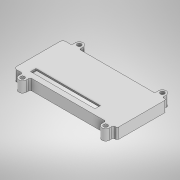
# Autodesk Inventor part: frontpackCOVER2
Saved by Autodesk Inventor 2021 (Build 250183000, 183)
## iProperties
Created: 2021-09-03
Part Number: frontpackCOVER2
Material: Generic
Document SubType Name: Modeling
Designer: perez
Density: 1 g/cm^3
Appearance: Default
Author: perez
Autodesk Inventor part; units mm, degrees
ref_plane "YZ Plane" through (0, 0, 0) normal (1, 0, 0) x (0, 1, 0)
ref_plane "XZ Plane" through (0, 0, 0) normal (0, 1, 0) x (-1, 0, 0)
ref_plane "XY Plane" through (0, 0, 0) normal (0, 0, 1) x (1, 0, 0)
sketch "Sketch1" plane through (0, 0, 0) normal (0, 1, 0) x (-1, 0, 0)
  line L0 (0, 0) -> (37, 0) construction
  line L1 (37, 0) -> (37, -30) construction
  line L2 (37, -30) -> (0, -30) construction
  line L3 (0, -30) -> (0, 0) construction
  line L4 (75.5, -6) -> (38, -6) construction
  line L5 (38, -6) -> (38, -24) construction
  line L6 (38, -24) -> (75.5, -24) construction
  line L7 (75.5, -24) -> (75.5, -6) construction
  line L8 (94, 0) -> (76.5, 0) construction
  line L9 (76.5, 0) -> (76.5, -28) construction
  line L10 (76.5, -28) -> (94, -28) construction
  line L11 (94, -28) -> (94, 0) construction
  line L12 (-1, 1) -> (117.5, 1)
  line L13 (117.5, 1) -> (117.5, -31)
  line L14 (117.5, -31) -> (-1, -31)
  line L15 (-1, -31) -> (-1, 1)
  line L16 (0, 0) -> (94, 0)
  line L17 (94, 0) -> (94, -30)
  line L18 (94, -30) -> (0, -30)
  line L19 (0, -30) -> (0, 0)
  line L20 (38, -8) -> (37, -8)
  line L21 (37, -8) -> (37, -22)
  line L22 (37, -22) -> (38, -22)
  line L23 (38, -22) -> (38, -8)
  line L24 (73.5, -6) -> (40, -6)
  line L25 (40, -6) -> (40, -5)
  line L26 (40, -5) -> (73.5, -5)
  line L27 (73.5, -5) -> (73.5, -6)
  line L28 (73.5, -24) -> (40, -24)
  line L29 (40, -24) -> (40, -25)
  line L30 (40, -25) -> (73.5, -25)
  line L31 (73.5, -25) -> (73.5, -24)
  line L32 (76.5, -8) -> (75.5, -8)
  line L33 (75.5, -8) -> (75.5, -22)
  line L34 (75.5, -22) -> (76.5, -22)
  line L35 (76.5, -22) -> (76.5, -8)
  line L36 (115, -31) -> (115, -33.5) construction
  line L37 (58.25, -31) -> (58.25, -33.5) construction
  line L38 (4, -31) -> (4, -33.5) construction
  line L39 (115, 1) -> (115, 3.5) construction
  line L40 (58.25, 1) -> (58.25, 3.5) construction
  line L41 (4, 1) -> (4, 3.5) construction
  circle A0 centre (115, -33.5) radius 2.5
  circle A1 centre (58.25, -33.5) radius 2.5
  circle A2 centre (4, -33.5) radius 2.5
  circle A3 centre (4, 3.5) radius 2.5
  circle A4 centre (58.25, 3.5) radius 2.5
  circle A5 centre (115, 3.5) radius 2.5
  line L42 (117.5, 1) -> (117.5, 3.5)
  line L43 (112.5, 3.5) -> (112.5, 1)
  line L44 (60.75, 3.5) -> (60.75, 1)
  line L45 (55.75, 3.5) -> (55.75, 1)
  line L46 (6.5, 3.5) -> (6.5, 1)
  line L47 (1.5, 3.5) -> (1.5, 1)
  line L48 (1.5, -33.5) -> (1.5, -31)
  line L49 (6.5, -33.5) -> (6.5, -31)
  line L50 (55.75, -33.5) -> (55.75, -31)
  line L51 (60.75, -33.5) -> (60.75, -31)
  line L52 (117.5, -33.5) -> (117.5, -31)
  line L53 (112.5, -33.5) -> (112.5, -31)
  circle A6 centre (115, -33.5) radius 1.55
  circle A7 centre (58.25, -33.5) radius 1.55
  circle A8 centre (4, -33.5) radius 1.55
  circle A9 centre (4, 3.5) radius 1.55
  circle A10 centre (58.25, 3.5) radius 1.55
  circle A11 centre (115, 3.5) radius 1.55
  line L54 (57.75, -30) -> (58.75, -30)
  line L55 (58.75, -30) -> (58.75, -25)
  line L56 (58.75, -25) -> (57.75, -25)
  line L57 (57.75, -25) -> (57.75, -30)
  line L58 (57.75, -5) -> (58.75, -5)
  line L59 (58.75, -5) -> (58.75, 0)
  line L60 (58.75, 0) -> (57.75, 0)
  line L61 (57.75, 0) -> (57.75, -5)
  line L62 (40, -25) -> (41, -25)
  line L63 (41, -25) -> (41, -30)
  line L64 (41, -30) -> (40, -30)
  line L65 (40, -30) -> (40, -25)
  line L66 (40, -5) -> (41, -5)
  line L67 (41, -5) -> (41, 0)
  line L68 (41, 0) -> (40, 0)
  line L69 (40, 0) -> (40, -5)
  line L70 (73.5, -5) -> (72.5, -5)
  line L71 (72.5, -5) -> (72.5, 0)
  line L72 (72.5, 0) -> (73.5, 0)
  line L73 (73.5, 0) -> (73.5, -5)
  line L74 (73.5, -25) -> (72.5, -25)
  line L75 (72.5, -25) -> (72.5, -30)
  line L76 (72.5, -30) -> (73.5, -30)
  line L77 (73.5, -30) -> (73.5, -25)
  dimension "d0" = 37
  dimension "d1" = 30
  dimension "d2" = 18
  dimension "d3" = 37.5
  dimension "d4" = 1
  dimension "d5" = 6
  dimension "d6" = 17.5
  dimension "d7" = 28
  dimension "d8" = 1
  dimension "d9" = 1
  dimension "d10" = 1
  dimension "d11" = 1
  dimension "d12" = 117.5
  dimension "d13" = 2
  dimension "d14" = 2
  dimension "d15" = 1
  dimension "d16" = 1
  dimension "d17" = 2
  dimension "d18" = 2
  dimension "d19" = 2
  dimension "d20" = 2
  dimension "d21" = 2.5
  dimension "d22" = 2.5
  dimension "d23" = 5
  dimension "d24" = 2.5
  dimension "d25" = 2.5
  dimension "d26" = 2.5
  dimension "d27" = 2.5
  dimension "d28" = 5
  dimension "d29" = 5
  dimension "d30" = 2.5
  dimension "d31" = 3.1
  dimension "d32" = 3.1
  dimension "d33" = 3.1
  dimension "d34" = 3.1
  dimension "d35" = 3.1
  dimension "d36" = 3.1
  dimension "d44" = 1
  dimension "d45" = 1
  dimension "d46" = 0.5
  dimension "d47" = 0
  dimension "d48" = 1
  dimension "d49" = 1
  dimension "d50" = 1
  dimension "d51" = 1
  constraints: 152 end point, 30 parallel, 24 point on line, 16 point on circle, 15 perpendicular, 14 horizontal, 12 centre point, 12 coincident, 12 vertical, 8 tangent, 22 other
  measures "d0" distance of L1.end L2.end
  measures "d1" distance of L0.end L1.end
  measures "d2" distance of L4.end L5.end
  measures "d3" distance of L5.end L6.end
  measures "d4" distance between parallel lines of L1 L5
  measures "d5" distance between parallel lines of L2 L6
  measures "d6" distance of L10.end L9.end
  measures "d7" distance of L9.end L8.end
  measures "d8" distance between parallel lines of L7 L9
  measures "d9" distance between parallel lines of L15 L3
  measures "d12" distance between parallel lines of L13 L3
  measures "d13" distance between parallel lines of L20 L4
  measures "d14" distance between parallel lines of L22 L6
  measures "d15" distance of L30.end L28.start
  measures "d16" distance of L26.end L24.start
  measures "d17" distance between parallel lines of L5 L25
  measures "d18" distance between parallel lines of L7 L27
  measures "d19" distance between parallel lines of L6 L34
  measures "d20" distance between parallel lines of L4 L32
  measures "d21" distance of L36.start L36.end
  measures "d22" distance between parallel lines of L13 L36
  measures "d23" distance between parallel lines of L15 L38
  measures "d24" distance of L37.start L37.end
  measures "d25" distance of L39.start L39.end
  measures "d26" distance of L40.start L40.end
  measures "d27" distance of L41.start L41.end
  measures "d28" diameter of A0
  measures "d29" diameter of A1
  measures "d30" distance of L38.start L38.end
  measures "d31" diameter of A6
  measures "d32" diameter of A7
  measures "d33" diameter of A8
  measures "d34" diameter of A9
  measures "d35" diameter of A10
  measures "d36" diameter of A11
  measures "d44" distance between parallel lines of L55 L57
  measures "d45" distance between parallel lines of L59 L61
  measures "d46" distance between parallel lines of L37 L57
  measures "d47" distance between parallel lines of L40 L37
  measures "d48" distance of L63.end L64.end
  measures "d49" distance of L68.end L67.end
  measures "d50" distance of L71.end L72.end
  measures "d51" distance of L76.end L75.end
extrude "Extrusion1" add sketch "Sketch1" along normal blind 7 contours L12 L13 L14 L15 | L47 A3 L12 | A3 L46 L12 | A3 | L14 A2 L48 | L14 L49 A2 | A2 | L45 A4 L12 | A4 L44 L12 | A4 | L14 A1 L50 | L14 L51 A1 | A1 | L43 A5 L12 | A5 L42 L12 | A5 | L14 A0 L53 | L14 L52 A0 | A0 | L16 L67 L26 L69 | L26 L27 L24 L25 | L65 L30 L63 L18 | L16 L59 L26 L61 | L29 L28 L31 L30 | L57 L30 L55 L18 | L16 L73 L26 L71 | L75 L30 L77 L18 | L23 L22 L21 L20 | L35 L34 L33 L32
sketch "Sketch2" plane through (0, 0, 0) normal (0, -1, 0) x (1, 0, 0)
  line L0 (-117.5, -33.5) -> (-117.5, 3.5) projected
  arc A0 (-117.5, -33.5) -> (-112.5, -33.5) centre (-115, -33.5) ccw projected
  line L1 (-112.5, -31) -> (-112.5, -33.5) projected
  line L2 (-60.75, -31) -> (-112.5, -31) projected
  line L3 (-60.75, -33.5) -> (-60.75, -31) projected
  arc A1 (-60.75, -33.5) -> (-55.75, -33.5) centre (-58.25, -33.5) ccw projected
  line L4 (-55.75, -31) -> (-55.75, -33.5) projected
  line L5 (-6.5, -31) -> (-55.75, -31) projected
  line L6 (-6.5, -33.5) -> (-6.5, -31) projected
  arc A2 (-6.5, -33.5) -> (-1.5, -33.5) centre (-4, -33.5) ccw projected
  line L7 (-1.5, -31) -> (-1.5, -33.5) projected
  line L8 (1, -31) -> (-1.5, -31) projected
  line L9 (1, 1) -> (1, -31) projected
  line L10 (-1.5, 1) -> (1, 1) projected
  line L11 (-1.5, 3.5) -> (-1.5, 1) projected
  arc A3 (-1.5, 3.5) -> (-6.5, 3.5) centre (-4, 3.5) ccw projected
  line L12 (-6.5, 1) -> (-6.5, 3.5) projected
  line L13 (-55.75, 1) -> (-6.5, 1) projected
  line L14 (-55.75, 3.5) -> (-55.75, 1) projected
  arc A4 (-55.75, 3.5) -> (-60.75, 3.5) centre (-58.25, 3.5) ccw projected
  line L15 (-60.75, 1) -> (-60.75, 3.5) projected
  line L16 (-112.5, 1) -> (-60.75, 1) projected
  line L17 (-112.5, 3.5) -> (-112.5, 1) projected
  arc A5 (-112.5, 3.5) -> (-117.5, 3.5) centre (-115, 3.5) ccw projected
  circle A6 centre (-58.25, 3.5) radius 1.55 projected
  circle A7 centre (-4, 3.5) radius 1.55 projected
  circle A8 centre (-4, -33.5) radius 1.55 projected
  circle A9 centre (-58.25, -33.5) radius 1.55 projected
  circle A10 centre (-115, 3.5) radius 1.55 projected
  circle A11 centre (-115, -33.5) radius 1.55 projected
  line L18 (-41, 0) -> (-57.75, 0) projected
  line L19 (0, -30) -> (0, 0) projected
  line L20 (-57.75, -30) -> (-41, -30) projected
  line L21 (-94, 0) -> (-94, -30) projected
  line L22 (-41, -5) -> (-41, 0) projected
  line L23 (-57.75, -5) -> (-41, -5) projected
  line L24 (-57.75, 0) -> (-57.75, -5) projected
  line L25 (-41, -30) -> (-41, -25) projected
  line L26 (-57.75, -25) -> (-57.75, -30) projected
  line L27 (-41, -25) -> (-57.75, -25) projected
  line L28 (-72.5, -25) -> (-72.5, -30) projected
  line L29 (-58.75, -25) -> (-72.5, -25) projected
  line L30 (-58.75, -30) -> (-58.75, -25) projected
  line L31 (-72.5, -30) -> (-58.75, -30) projected
  line L32 (-72.5, 0) -> (-72.5, -5) projected
  line L33 (-58.75, 0) -> (-72.5, 0) projected
  line L34 (-58.75, -5) -> (-58.75, 0) projected
  line L35 (-72.5, -5) -> (-58.75, -5) projected
  line L36 (-73.5, 0) -> (-94, 0) projected
  line L37 (-73.5, -6) -> (-73.5, 0) projected
  line L38 (-40, -6) -> (-73.5, -6) projected
  line L39 (-40, 0) -> (-40, -6) projected
  line L40 (0, 0) -> (-40, 0) projected
  line L41 (-40, -30) -> (0, -30) projected
  line L42 (-40, -24) -> (-40, -30) projected
  line L43 (-73.5, -24) -> (-40, -24) projected
  line L44 (-73.5, -30) -> (-73.5, -24) projected
  line L45 (-94, -30) -> (-73.5, -30) projected
extrude "Extrusion2" add sketch "Sketch2" along normal blind 1 contours L0 A5 L17 L16 L15 A4 L14 L13 L12 A3 L11 L10 L9 L8 L7 A2 L6 L5 L4 A1 L3 L2 L1 A0 | L22 L23 L24 L18 | L41 L42 L43 L44 L45 L21 L36 L37 L38 L39 L40 L19 | L26 L27 L25 L20 | L29 L30 L31 L28 | L33 L34 L35 L32
fillet "Fillet2" radius 1 32 edges at (-73.5, 3.5, -6) (-73.5, 3.5, -24) (-40, 3.5, -24) (1, 3, -31) (-1.5, 3, -31) (1, 3, 1) (-55.75, 3, -31) (-1.5, 3, 1) (-55.75, 3, 1) (-112.5, 3, 1) (-112.5, 3, -31) (-60.75, 3, -31) (-6.5, 3, -31) (-60.75, 3, 1) (-6.5, 3, 1) (-40, 3.5, -6) (-72.5, 3.5, 0) (-57.75, 3.5, 0) (-72.5, 3.5, -25) (-57.75, 3.5, -25) (-41, 3.5, -25) (-58.75, 3.5, -25) (-41, 3.5, 0) (-58.75, 3.5, 0) (-72.5, 3.5, -30) (-57.75, 3.5, -30) (-57.75, 3.5, -5) (-72.5, 3.5, -5) (-41, 3.5, -5) (-58.75, 3.5, -5) (-58.75, 3.5, -30) (-41, 3.5, -30)
sketch "Sketch5" plane through (0, 7, 0) normal (0, 1, 0) x (1, 0, 0)
  line L0 (-120.447, 38.9055) -> (3.6698, 38.9055)
  line L1 (3.6698, 38.9055) -> (3.6698, -10.7705)
  line L2 (3.6698, -10.7705) -> (-120.447, -10.7705)
  line L3 (-120.447, -10.7705) -> (-120.447, 38.9055)
  point P0 (0, 0)
  constraints: 8 end point, 2 parallel, 1 horizontal, 1 perpendicular
extrude "Extrusion5" cut sketch "Sketch5" against normal blind 7
sketch "Sketch13" plane through (0, 0, 0) normal (0, 1, 0) x (1, 0, 0)
  line L0 (-64.5, 29) -> (-1, 29)
  line L1 (-1, 29) -> (-1, 1)
  line L2 (-1, 1) -> (-64.5, 1)
  line L3 (-64.5, 1) -> (-64.5, 29)
  line L4 (1, 30) -> (1, 0) projected
  line L5 (-54.75, 31) -> (-7.5, 31) projected
  line L6 (-7.5, -1) -> (-54.75, -1) projected
  line L7 (-117.5, -3.5) -> (-117.5, 33.5) projected
  line L8 (-77.5, 28.5) -> (-67.5, 28.5)
  line L9 (-67.5, 28.5) -> (-67.5, 21.5)
  line L10 (-67.5, 21.5) -> (-77.5, 21.5)
  line L11 (-77.5, 21.5) -> (-77.5, 28.5)
  line L12 (-77.5, 11) -> (-67.5, 11)
  line L13 (-67.5, 11) -> (-67.5, 4)
  line L14 (-67.5, 4) -> (-77.5, 4)
  line L15 (-77.5, 4) -> (-77.5, 11)
  line L16 (-111.5, 31) -> (-61.75, 31) projected
  line L17 (-61.75, -1) -> (-111.5, -1) projected
  point P0 (0, 0)
  point P1 (-77.5, 25)
  point P2 (-77.5, 7.5)
  point P3 (-67.5, 25)
  point P4 (-67.5, 7.5)
  dimension "d114" = 2
  dimension "d115" = 2
  dimension "d116" = 2
  dimension "d117" = 53
  dimension "d118" = 50
  dimension "d119" = 10
  dimension "d120" = 2.5
  dimension "d121" = 5
  dimension "d122" = 12
  dimension "d123" = 9.5
  constraints: 24 end point, 6 parallel, 4 midpoint, 3 horizontal, 3 perpendicular, 2 vertical alignment, 1 point on line
  measures "d114" distance between parallel lines of L4 L1
  measures "d115" distance between parallel lines of L0 L5
  measures "d116" distance between parallel lines of L6 L2
  measures "d117" distance between parallel lines of L3 L7
  measures "d118" distance between parallel lines of L7 L9
  measures "d119" distance of L8.start L8.end
  measures "d120" distance between parallel lines of L16 L8
  measures "d121" distance between parallel lines of L17 L14
  measures "d122" distance between parallel lines of L17 L12
  measures "d123" distance between parallel lines of L10 L16
extrude "Extrusion15" cut sketch "Sketch13" against normal through all
fillet "Fillet4" radius 2 12 edges at (-64.5, -0.5, -29) (-77.5, -0.5, -28.5) (-77.5, -0.5, -11) (-1, -0.5, -29) (-1, -0.5, -1) (-67.5, -0.5, -4) (-67.5, -0.5, -21.5) (-64.5, -0.5, -1) (-77.5, -0.5, -4) (-77.5, -0.5, -21.5) (-67.5, -0.5, -28.5) (-67.5, -0.5, -11)
sketch "Sketch14" plane through (0, 0, 0) normal (0, 1, 0) x (1, 0, 0)
  line L0 (-122.4495, 38.8167) -> (-66.5, 38.8167)
  line L1 (-66.5, 38.8167) -> (-66.5, -7.5012)
  line L2 (-66.5, -7.5012) -> (-122.4495, -7.5012)
  line L3 (-122.4495, -7.5012) -> (-122.4495, 38.8167)
  line L4 (-64.5, 3) -> (-64.5, 27) projected
  point P0 (0, 0)
  dimension "d127" = 2
  constraints: 8 end point, 2 parallel, 1 horizontal, 1 perpendicular
  measures "d127" distance between parallel lines of L1 L4
extrude "Extrusion16" cut sketch "Sketch14" against normal blind 10
fillet "Fillet5" radius 2 2 edges at (-66.5, -0.5, 1) (-66.5, -0.5, -31)
sketch "Sketch15" plane through (0, -1, 0) normal (0, -1, 0) x (1, 0, 0)
  point P0 (0, 0)
sketch "Sketch16" plane through (0, 0, 0) normal (0, 1, 0) x (1, 0, 0)
  arc A0 (-64.5, 31) -> (-66.5, 29) centre (-64.5, 29) ccw projected
  line L0 (-66.5, 29) -> (-66.5, 1) projected
  arc A1 (-66.5, 1) -> (-64.5, -1) centre (-64.5, 1) ccw projected
  line L1 (-61.75, -1) -> (-64.5, -1) projected
  arc A2 (-60.75, -2) -> (-61.75, -1) centre (-61.75, -2) ccw projected
  line L2 (-60.75, -3.5) -> (-60.75, -2) projected
  arc A3 (-60.75, -3.5) -> (-55.75, -3.5) centre (-58.25, -3.5) ccw projected
  line L3 (-55.75, -2) -> (-55.75, -3.5) projected
  arc A4 (-54.75, -1) -> (-55.75, -2) centre (-54.75, -2) ccw projected
  line L4 (-7.5, -1) -> (-54.75, -1) projected
  arc A5 (-6.5, -2) -> (-7.5, -1) centre (-7.5, -2) ccw projected
  line L5 (-6.5, -3.5) -> (-6.5, -2) projected
  arc A6 (-6.5, -3.5) -> (-1.5, -3.5) centre (-4, -3.5) ccw projected
  line L6 (-1.5, -2) -> (-1.5, -3.5) projected
  arc A7 (-0.5, -1) -> (-1.5, -2) centre (-0.5, -2) ccw projected
  line L7 (0, -1) -> (-0.5, -1) projected
  arc A8 (0, -1) -> (1, 0) centre (0, 0) ccw projected
  line L8 (1, 30) -> (1, 0) projected
  arc A9 (1, 30) -> (0, 31) centre (0, 30) ccw projected
  line L9 (-0.5, 31) -> (0, 31) projected
  arc A10 (-1.5, 32) -> (-0.5, 31) centre (-0.5, 32) ccw projected
  line L10 (-1.5, 33.5) -> (-1.5, 32) projected
  arc A11 (-1.5, 33.5) -> (-6.5, 33.5) centre (-4, 33.5) ccw projected
  line L11 (-6.5, 32) -> (-6.5, 33.5) projected
  arc A12 (-7.5, 31) -> (-6.5, 32) centre (-7.5, 32) ccw projected
  line L12 (-54.75, 31) -> (-7.5, 31) projected
  arc A13 (-55.75, 32) -> (-54.75, 31) centre (-54.75, 32) ccw projected
  line L13 (-55.75, 33.5) -> (-55.75, 32) projected
  arc A14 (-55.75, 33.5) -> (-60.75, 33.5) centre (-58.25, 33.5) ccw projected
  line L14 (-60.75, 32) -> (-60.75, 33.5) projected
  arc A15 (-61.75, 31) -> (-60.75, 32) centre (-61.75, 32) ccw projected
  line L15 (-64.5, 31) -> (-61.75, 31) projected
  circle A16 centre (-58.25, 33.5) radius 1.55 projected
  circle A17 centre (-4, 33.5) radius 1.55 projected
  circle A18 centre (-4, -3.5) radius 1.55 projected
  circle A19 centre (-58.25, -3.5) radius 1.55 projected
  line L16 (-1, 27) -> (-1, 3) projected
  arc A20 (-3, 1) -> (-1, 3) centre (-3, 3) ccw projected
  line L17 (-3, 1) -> (-62.5, 1) projected
  arc A21 (-64.5, 3) -> (-62.5, 1) centre (-62.5, 3) ccw projected
  line L18 (-64.5, 3) -> (-64.5, 27) projected
  arc A22 (-62.5, 29) -> (-64.5, 27) centre (-62.5, 27) ccw projected
  line L19 (-62.5, 29) -> (-3, 29) projected
  arc A23 (-1, 27) -> (-3, 29) centre (-3, 27) ccw projected
  point P0 (0, 0)
extrude "Extrusion17" add sketch "Sketch16" along normal blind 5
sketch "Sketch17" plane through (0, 5, 0) normal (0, 1, 0) x (1, 0, 0)
  arc A0 (-64.5, 31) -> (-66.5, 29) centre (-64.5, 29) ccw projected
  line L0 (-66.5, 29) -> (-66.5, 1) projected
  arc A1 (-66.5, 1) -> (-64.5, -1) centre (-64.5, 1) ccw projected
  line L1 (-64.5, -1) -> (-61.75, -1) projected
  arc A2 (-60.75, -2) -> (-61.75, -1) centre (-61.75, -2) ccw projected
  line L2 (-60.75, -2) -> (-60.75, -3.5) projected
  arc A3 (-60.75, -3.5) -> (-55.75, -3.5) centre (-58.25, -3.5) ccw projected
  line L3 (-55.75, -3.5) -> (-55.75, -2) projected
  arc A4 (-54.75, -1) -> (-55.75, -2) centre (-54.75, -2) ccw projected
  line L4 (-54.75, -1) -> (-7.5, -1) projected
  arc A5 (-6.5, -2) -> (-7.5, -1) centre (-7.5, -2) ccw projected
  line L5 (-6.5, -2) -> (-6.5, -3.5) projected
  arc A6 (-6.5, -3.5) -> (-1.5, -3.5) centre (-4, -3.5) ccw projected
  line L6 (-1.5, -3.5) -> (-1.5, -2) projected
  arc A7 (-0.5, -1) -> (-1.5, -2) centre (-0.5, -2) ccw projected
  line L7 (-0.5, -1) -> (0, -1) projected
  arc A8 (0, -1) -> (1, 0) centre (0, 0) ccw projected
  line L8 (1, 0) -> (1, 30) projected
  arc A9 (1, 30) -> (0, 31) centre (0, 30) ccw projected
  line L9 (0, 31) -> (-0.5, 31) projected
  arc A10 (-1.5, 32) -> (-0.5, 31) centre (-0.5, 32) ccw projected
  line L10 (-1.5, 32) -> (-1.5, 33.5) projected
  arc A11 (-1.5, 33.5) -> (-6.5, 33.5) centre (-4, 33.5) ccw projected
  line L11 (-6.5, 33.5) -> (-6.5, 32) projected
  arc A12 (-7.5, 31) -> (-6.5, 32) centre (-7.5, 32) ccw projected
  line L12 (-7.5, 31) -> (-54.75, 31) projected
  arc A13 (-55.75, 32) -> (-54.75, 31) centre (-54.75, 32) ccw projected
  line L13 (-55.75, 32) -> (-55.75, 33.5) projected
  arc A14 (-55.75, 33.5) -> (-60.75, 33.5) centre (-58.25, 33.5) ccw projected
  line L14 (-60.75, 33.5) -> (-60.75, 32) projected
  arc A15 (-61.75, 31) -> (-60.75, 32) centre (-61.75, 32) ccw projected
  line L15 (-61.75, 31) -> (-64.5, 31) projected
  line L16 (-62.5, 29) -> (-3, 29) projected
  arc A16 (-1, 27) -> (-3, 29) centre (-3, 27) ccw projected
  line L17 (-1, 27) -> (-1, 3) projected
  arc A17 (-3, 1) -> (-1, 3) centre (-3, 3) ccw projected
  line L18 (-3, 1) -> (-62.5, 1) projected
  arc A18 (-64.5, 3) -> (-62.5, 1) centre (-62.5, 3) ccw projected
  line L19 (-64.5, 3) -> (-64.5, 27) projected
  arc A19 (-62.5, 29) -> (-64.5, 27) centre (-62.5, 27) ccw projected
  circle A20 centre (-58.25, -3.5) radius 1.55 projected
  circle A21 centre (-4, -3.5) radius 1.55 projected
  circle A22 centre (-4, 33.5) radius 1.55 projected
  circle A23 centre (-58.25, 33.5) radius 1.55 projected
  point P0 (0, 0)
extrude "Extrusion18" add sketch "Sketch17" along normal blind 1 contours L15 A15 L14 A14 L13 A13 L12 A12 L11 A11 L10 A10 L9 A9 L8 A8 L7 A7 L6 A6 L5 A5 L4 A4 L3 A3 L2 A2 L1 A1 L0 A0 | L16 A16 L17 A17 L18 A18 L19 A19
sketch "Sketch18" plane through (0, 6, 0) normal (0, 1, 0) x (1, 0, 0)
  line L0 (-59, 6) -> (-17, 6)
  line L1 (-17, 6) -> (-17, 2.5)
  line L2 (-17, 2.5) -> (-59, 2.5)
  line L3 (-59, 2.5) -> (-59, 6)
  circle A0 centre (-4, -3.5) radius 1.55 projected
  circle A1 centre (-58.25, -3.5) radius 1.55 projected
  circle A2 centre (-4, 33.5) radius 1.55 projected
  line L4 (-54.75, -1) -> (-7.5, -1) projected
  line L5 (-66.5, 29) -> (-66.5, 1) projected
  line L6 (1, 0) -> (1, 30) projected
  point P0 (0, 0)
  dimension "d147" = 3.5
  dimension "d148" = 7
  dimension "d149" = 7.5
  dimension "d150" = 18
  constraints: 8 end point, 2 parallel, 1 horizontal, 1 perpendicular
  measures "d147" distance between parallel lines of L4 L2
  measures "d148" distance between parallel lines of L4 L0
  measures "d149" distance between parallel lines of L5 L3
  measures "d150" distance between parallel lines of L6 L1
extrude "Extrusion20" cut sketch "Sketch18" against normal blind 10 contours L0 L1 L2 L3
sketch "Sketch20" plane through (0, 6, 0) normal (0, 1, 0) x (1, 0, 0)
  circle A0 centre (-58.25, 33.5) radius 1.55 projected
  circle A1 centre (-4, 33.5) radius 1.55 projected
  circle A2 centre (-4, -3.5) radius 1.55 projected
  circle A3 centre (-58.25, -3.5) radius 1.55 projected
  circle A4 centre (-58.25, 33.5) radius 1.35
  circle A5 centre (-4, 33.5) radius 1.35
  circle A6 centre (-58.25, -3.5) radius 1.35
  circle A7 centre (-4, -3.5) radius 1.35
  point P0 (0, 0)
  dimension "d153" = 2.7
  dimension "d154" = 2.7
  dimension "d155" = 2.7
  dimension "d156" = 2.7
  constraints: 4 centre point, 4 coincident
  measures "d153" diameter of A4
  measures "d154" diameter of A5
  measures "d155" diameter of A6
  measures "d156" diameter of A7
extrude "Extrusion21" add sketch "Sketch20" against normal up to surface (7 mm away)
body "Solid1"
